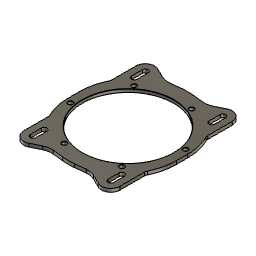
Motor_Base_Plate_Top v5 (Autodesk Fusion 360 archive; units mm, degrees)
design "Motor_Base_Plate_Top v5" references "Forged Hexagon Socket Head Cap Screw ANSI B18.3.1M - M4x0.7 x 6 Steel Grade 2 Plain"
Autodesk Fusion 360 part; units mm, degrees
sketch "Sketch1" plane through (0, 0, 0) normal (0, 0, 1) x (1, 0, 0)
  line L0 (0, 0) -> (42.0984, 0) construction
  line L1 (0, 2.5) -> (0, 20)
  line L2 (20, 0) -> (2.5, 0)
  line L3 (43.5453, 45.7571) -> (43.5453, 28.6506)
  arc A0 (32.6927, 46.2539) -> (32.6429, 45.7571) centre (35.1429, 45.7571) ccw
  line L4 (-32.6429, 45.7571) -> (-32.6429, 40.7571)
  arc A1 (-32.6429, 45.7571) -> (-32.7077, 46.3226) centre (-35.1429, 45.7571) ccw
  line L5 (-43.5453, 45.7571) -> (-43.5453, 28.6506)
  line L6 (16.6515, 53.2283) -> (16.6515, 59.0493) construction
  line L7 (-15.557, 53.706) -> (-15.557, 59.527) construction
  line L8 (0, 0) -> (45, 0) construction
  arc A2 (-41.8537, 25.4807) -> (-42.1265, 25.0272) centre (0, 0) ccw
  arc A3 (4.0267, 61.4469) -> (-4.7848, 61.3754) centre (-0.036, 19.1415) ccw
  arc A4 (43.4103, 49.257) -> (33.6006, 59.0168) centre (35.1429, 50.7571) ccw
  line L9 (16.6515, 58.2283) -> (16.6515, 64.0493) construction
  arc A5 (28.1023, 59.5419) -> (33.6006, 59.0168) centre (31.7651, 68.8469) ccw
  arc A6 (14.9315, 52.7652) -> (22.9245, 54.1858) centre (16.401, 67.693) ccw
  line L10 (-22.9245, 54.1858) -> (-31.3596, 58.2597)
  arc A7 (49, 5) -> (41.8537, 30.4807) centre (0, 5) ccw
  line L11 (43.5453, 50.7571) -> (43.5453, 28.6506)
  line L12 (14.9315, 52.7652) -> (5.4274, 53.7007)
  line L13 (-41.2861, 38.5638) -> (-43.4103, 49.257)
  arc A8 (-9.7818, 62.096) -> (-4.7848, 61.3754) centre (-5.9022, 71.3127) ccw
  line L14 (-14.9315, 52.7652) -> (-5.4274, 53.7007)
  arc A9 (-37.6429, 40.7571) -> (-32.6429, 40.7571) centre (-35.1429, 40.7571) ccw
  circle A10 centre (-15.557, 58.706) radius 1.5
  line L15 (-43.5453, 50.7571) -> (-43.5453, 28.6506)
  arc A11 (-44.0504, 26.4608) -> (-43.5453, 28.6506) centre (-48.5453, 28.6506) ccw
  arc A12 (-32.6429, 50.7571) -> (-37.6429, 50.7571) centre (-35.1429, 50.7571) ccw
  line L16 (-19.3563, 63.0202) -> (-28.095, 59.5544)
  arc A13 (-33.6082, 59.0182) -> (-28.095, 59.5544) centre (-31.7817, 68.85) ccw
  line L17 (-7.2407, 61.0264) -> (-0.4717, 58.2301) construction
  arc A14 (-11.79, 62.9413) -> (-19.3563, 63.0202) centre (-15.6696, 53.7246) ccw
  arc A15 (43.5453, 28.6506) -> (44.0504, 26.4608) centre (48.5453, 28.6506) ccw
  line L18 (-11.79, 62.9413) -> (-9.7818, 62.096)
  line L19 (41.2861, 38.5638) -> (43.4103, 49.257)
  arc A16 (-7.2407, 61.0264) -> (6.4194, 61.1484) centre (-0.036, 19.1415) ccw construction
  line L20 (-32.6429, 50.7571) -> (-32.6429, 45.7571)
  arc A17 (-22.9245, 54.1858) -> (-14.9315, 52.7652) centre (-16.401, 67.693) ccw
  arc A18 (41.2861, 38.5638) -> (41.8537, 30.4807) centre (56.0268, 35.5374) ccw
  line L21 (-15.557, 58.706) -> (-15.557, 64.527) construction
  line L22 (11.1293, 63.1457) -> (8.8867, 62.1947)
  arc A19 (4.0267, 61.4469) -> (8.8867, 62.1947) centre (4.9826, 71.4011) ccw
  line L23 (6.4194, 61.1484) -> (-0.4717, 58.2301) construction
  arc A20 (43.4103, 49.257) -> (31.3596, 58.2597) centre (35.1429, 50.7571) ccw
  line L24 (-37.6429, 50.7571) -> (-37.6429, 40.7571)
  arc A21 (-33.6006, 59.0168) -> (-43.4103, 49.257) centre (-35.1429, 50.7571) ccw
  arc A22 (-41.8537, 30.4807) -> (-41.2861, 38.5638) centre (-56.0268, 35.5374) ccw
  arc A23 (-31.3596, 58.2597) -> (-43.4103, 49.257) centre (-35.1429, 50.7571) ccw
  arc A24 (18.6963, 63.2444) -> (11.1293, 63.1457) centre (15.0335, 53.9393) ccw
  arc A25 (5.4274, 53.7007) -> (-5.4274, 53.7007) centre (0, 5) ccw
  circle A26 centre (16.6515, 58.2283) radius 1.5
  arc A27 (-41.8537, 30.4807) -> (-49, 5) centre (0, 5) ccw
  line L25 (18.6963, 63.2444) -> (28.1023, 59.5419)
  line L26 (22.9245, 54.1858) -> (31.3596, 58.2597)
  arc A28 (-33.6006, 54.0168) -> (-33.6082, 54.0182) centre (-35.1429, 45.7571) ccw
  line L27 (32.6429, 45.7571) -> (32.6429, 40.7571)
  line L28 (32.6429, 50.7571) -> (32.6429, 45.7571)
  line L29 (37.6429, 50.7571) -> (37.6429, 40.7571)
  arc A29 (37.6429, 50.7571) -> (32.6429, 50.7571) centre (35.1429, 50.7571) ccw
  arc A30 (32.6429, 40.7571) -> (37.6429, 40.7571) centre (35.1429, 40.7571) ccw
  arc A31 (-5.4274, -53.7007) -> (5.4274, -53.7007) centre (0, -5) ccw
  arc A32 (22.9245, -54.1858) -> (14.9315, -52.7652) centre (16.401, -67.693) ccw
  arc A33 (32.6429, -45.7571) -> (32.6927, -46.2539) centre (35.1429, -45.7571) ccw
  line L30 (-15.557, -53.706) -> (-15.557, -59.527) construction
  arc A34 (31.3596, -58.2597) -> (43.4103, -49.257) centre (35.1429, -50.7571) ccw
  line L31 (6.4194, -61.1484) -> (-0.4717, -58.2301) construction
  circle A35 centre (16.6515, -58.2283) radius 1.5
  arc A36 (-49, -5) -> (-41.8537, -30.4807) centre (0, -5) ccw
  arc A37 (32.6429, -50.7571) -> (37.6429, -50.7571) centre (35.1429, -50.7571) ccw
  arc A38 (-42.1265, -25.0272) -> (-41.8537, -25.4807) centre (0, 0) ccw
  line L32 (-11.79, -62.9413) -> (-9.7818, -62.096)
  arc A39 (8.8867, -62.1947) -> (4.0267, -61.4469) centre (4.9826, -71.4011) ccw
  arc A40 (-41.2861, -38.5638) -> (-41.8537, -30.4807) centre (-56.0268, -35.5374) ccw
  line L33 (11.1293, -63.1457) -> (8.8867, -62.1947)
  arc A41 (-43.5453, -28.6506) -> (-44.0504, -26.4608) centre (-48.5453, -28.6506) ccw
  line L34 (-22.9245, -54.1858) -> (-31.3596, -58.2597)
  arc A42 (-19.3563, -63.0202) -> (-11.79, -62.9413) centre (-15.6696, -53.7246) ccw
  arc A43 (-33.6082, -54.0182) -> (-33.6006, -54.0168) centre (-35.1429, -45.7571) ccw
  arc A44 (-37.6429, -50.7571) -> (-32.6429, -50.7571) centre (-35.1429, -50.7571) ccw
  arc A45 (-4.7848, -61.3754) -> (4.0267, -61.4469) centre (-0.036, -19.1415) ccw
  arc A46 (-32.7077, -46.3226) -> (-32.6429, -45.7571) centre (-35.1429, -45.7571) ccw
  line L35 (-32.6429, -45.7571) -> (-32.6429, -40.7571)
  line L36 (22.9245, -54.1858) -> (31.3596, -58.2597)
  line L37 (-15.557, -58.706) -> (-15.557, -64.527) construction
  line L38 (32.6429, -45.7571) -> (32.6429, -40.7571)
  line L39 (32.6429, -50.7571) -> (32.6429, -45.7571)
  line L40 (-43.5453, -45.7571) -> (-43.5453, -28.6506)
  line L41 (37.6429, -50.7571) -> (37.6429, -40.7571)
  line L42 (14.9315, -52.7652) -> (5.4274, -53.7007)
  arc A47 (-14.9315, -52.7652) -> (-22.9245, -54.1858) centre (-16.401, -67.693) ccw
  line L43 (43.5453, -45.7571) -> (43.5453, -28.6506)
  line L44 (-43.5453, -50.7571) -> (-43.5453, -28.6506)
  arc A48 (-43.5453, -23.6506) -> (-44.0504, -21.4608) centre (-48.5453, -23.6506) ccw
  line L45 (41.2861, -38.5638) -> (43.4103, -49.257)
  arc A49 (-28.095, -59.5544) -> (-33.6082, -59.0182) centre (-31.7817, -68.85) ccw
  arc A50 (-4.7848, -61.3754) -> (-9.7818, -62.096) centre (-5.9022, -71.3127) ccw
  line L46 (20, 0) -> (2.5, 0)
  line L47 (16.6515, -53.2283) -> (16.6515, -59.0493) construction
  line L48 (18.6963, -63.2444) -> (28.1023, -59.5419)
  arc A51 (33.6006, -59.0168) -> (43.4103, -49.257) centre (35.1429, -50.7571) ccw
  line L49 (-7.2407, -61.0264) -> (-0.4717, -58.2301) construction
  arc A52 (41.8537, -30.4807) -> (49, -5) centre (0, -5) ccw
  arc A53 (-43.4103, -49.257) -> (-33.6006, -59.0168) centre (-35.1429, -50.7571) ccw
  line L50 (16.6515, -58.2283) -> (16.6515, -64.0493) construction
  arc A54 (44.0504, -26.4608) -> (43.5453, -28.6506) centre (48.5453, -28.6506) ccw
  circle A55 centre (-15.557, -58.706) radius 1.5
  line L51 (-41.2861, -38.5638) -> (-43.4103, -49.257)
  arc A56 (41.8537, -30.4807) -> (41.2861, -38.5638) centre (56.0268, -35.5374) ccw
  arc A57 (33.6006, -59.0168) -> (28.1023, -59.5419) centre (31.7651, -68.8469) ccw
  line L52 (-19.3563, -63.0202) -> (-28.095, -59.5544)
  line L53 (-37.6429, -50.7571) -> (-37.6429, -40.7571)
  arc A58 (6.4194, -61.1484) -> (-7.2407, -61.0264) centre (-0.036, -19.1415) ccw construction
  line L54 (-14.9315, -52.7652) -> (-5.4274, -53.7007)
  line L55 (-32.6429, -50.7571) -> (-32.6429, -45.7571)
  arc A59 (37.6429, -40.7571) -> (32.6429, -40.7571) centre (35.1429, -40.7571) ccw
  arc A60 (-43.4103, -49.257) -> (-31.3596, -58.2597) centre (-35.1429, -50.7571) ccw
  arc A61 (-32.6429, -40.7571) -> (-37.6429, -40.7571) centre (-35.1429, -40.7571) ccw
  line L56 (43.5453, -50.7571) -> (43.5453, -28.6506)
  arc A62 (11.1293, -63.1457) -> (18.6963, -63.2444) centre (15.0335, -53.9393) ccw
  line L57 (49, 5) -> (49, -5)
  line L58 (-49, -5) -> (-49, 5)
  circle A63 centre (0, 0) radius 45 construction
  line L59 (0, 0) -> (45, 0) construction
  circle A64 centre (0, 0) radius 41.25
  line L60 (0, 0) -> (45, 0) construction
  line L61 (0, 0) -> (45, 0) construction
  line L62 (0, 0) -> (45, 0) construction
  line L63 (0, 0) -> (-15.3909, -42.2862) construction
  line L64 (0, 0) -> (45, 0) construction
  circle A65 centre (-15.3909, -42.2862) radius 2
  circle A66 centre (28.9254, -34.472) radius 2
  circle A67 centre (44.3163, 7.8142) radius 2
  circle A68 centre (15.3909, 42.2862) radius 2
  circle A69 centre (-28.9254, 34.472) radius 2
  circle A70 centre (-44.3163, -7.8142) radius 2
  point P0 (0, 5)
  point P1 (0, 5)
  point P2 (0, -5)
  point P3 (0, -2.5)
  point P4 (0, -5)
  point P5 (42.0984, 0)
  point P6 (0, -20)
  point P7 (45, 0)
  dimension "d52" = 5.821
  dimension "d53" = 5.821
  dimension "d60" = 85
  dimension "d61" = 3
  dimension "d62" = 5.821
  dimension "d63" = 5.821
  dimension "d64" = 10
  dimension "d66" = 90
  dimension "d71" = 82.5
  dimension "d121" = 110
  dimension "d122" = 4
  dimension "d124" = 360
  constraint coincident L0.start L8.start
  constraint horizontal L0
  constraint symmetric L1 L3.start L5.start
  constraint vertical L6
  constraint vertical L7
  constraint horizontal L8
  constraint tangent L14 A17
  constraint concentric A25 A27
  constraint coincident L9.start A16
  constraint coincident A10.centre A16
  constraint coincident L9.start A26.centre
  constraint vertical L9
  constraint coincident A10.centre L21.start
  constraint vertical L21
  constraint concentric A3 A16
  constraint coincident A20.end L25
  constraint coincident A20.end A4
  constraint tangent A4 A5
  constraint tangent A5 L25
  constraint coincident L9.end L25
  constraint tangent A24 L25
  constraint tangent L22 A24
  constraint equal A5 A24
  constraint coincident A16.end L22
  constraint tangent L22 A19
  constraint tangent A3 A19
  constraint equal A5 A19
  constraint coincident L17.start L18
  constraint coincident L17.start A3
  constraint tangent A3 A8
  constraint tangent A8 L18
  constraint equal A5 A8
  constraint coincident L21.end L16
  constraint coincident L21.end L18
  constraint tangent L16 A14
  constraint tangent A14 L18
  constraint equal A5 A14
  constraint tangent L16 A13
  constraint equal A5 A13
  constraint coincident A16 A2.end
  constraint coincident A16 A1.end
  constraint coincident A16 A0.start
  constraint symmetric L1 L4.start A0.end
  constraint symmetric L1 A12.start L28.start
  constraint symmetric L1 A12.end L29.start
  constraint symmetric L1 L4.end L27.end
  constraint symmetric L1 A9.start L29.end
  constraint symmetric L1 A9 A30
  constraint symmetric L1 A12 A29
  constraint symmetric L8.start L0 A2.centre
  constraint symmetric P5 L0 L0.end
  constraint symmetric L0 L8.start A2.centre
  constraint symmetric L0 A2.start A38.end
  constraint symmetric L0 L1.start P3
  constraint symmetric L0 L1.end P6
  constraint symmetric L0 L2.start L46.start
  constraint symmetric L0 L2.end L46.end
  constraint symmetric L0 L3.start L43.start
  constraint symmetric L0 A0.end A33.start
  constraint symmetric L0 A0 A33
  constraint symmetric L0 L4.start A46.end
  constraint symmetric L0 A1 A46
  constraint symmetric L0 L5.start L40.start
  constraint symmetric L0 L6.start L47.start
  constraint symmetric L0 L6.end L47.end
  constraint symmetric L0 L7.start L30.start
  constraint symmetric L0 L7.end L30.end
  constraint symmetric L0 A28.end A43.start
  constraint symmetric L0 A28.start A43.end
  constraint symmetric L0 P7 L8.end
  constraint symmetric L0 A2 A38
  constraint symmetric L0 L9.end L50.end
  constraint symmetric L0 P1 P4
  constraint symmetric L0 L12.end A31.end
  constraint symmetric L0 L13.start A40.start
  constraint symmetric L0 A15.end A54.start
  constraint symmetric L0 A4.end A51.start
  constraint symmetric L0 A4.start A34.end
  constraint symmetric L0 A12.start A44.end
  constraint symmetric L0 A12.end A44.start
  constraint symmetric L0 L9.start A35.centre
  constraint symmetric L0 L4.end L35.end
  constraint symmetric L0 L22.start L33.start
  constraint symmetric L0 A16.end L31.start
  constraint symmetric L0 L19.start L45.start
  constraint symmetric L0 A20.end A34.start
  constraint symmetric L0 A7.end A52.start
  constraint symmetric L0 A3.start A39.end
  constraint symmetric L0 L22.end A39.start
  constraint symmetric L0 A6.end A32.start
  constraint symmetric L0 L10.start L34.start
  constraint symmetric L0 A24.start L48.start
  constraint symmetric L0 L15.start L44.start
  constraint symmetric L0 A3.end A45.start
  constraint symmetric L0 L10.end L34.end
  constraint symmetric L0 L5.end A41.start
  constraint symmetric L0 L13.end A53.start
  constraint symmetric L0 A7.start A52.end
  constraint symmetric L0 A5.start L48.end
  constraint symmetric L0 A11.start A41.end
  constraint symmetric L0 L14.end A31.start
  constraint symmetric L0 L17.start L49.start
  constraint symmetric L0 A21.start A53.end
  constraint symmetric L0 L21.end L37.end
  constraint symmetric L0 A10.centre L37.start
  constraint symmetric L0 L3.end L43.end
  constraint symmetric L0 L16.start A42.start
  constraint symmetric L0 A8.start L32.end
  constraint symmetric L0 A14.start L32.start
  constraint symmetric L0 A9.start L53.end
  constraint symmetric L0 A22.start A36.end
  constraint symmetric L0 A6.start A32.end
  constraint symmetric L0 L16.end A49.start
  constraint symmetric L0 L11.start L56.start
  constraint symmetric L0 A27.end A36.start
  constraint symmetric L0 L14.start A47.start
  constraint symmetric L0 L17.end L31.end
  constraint symmetric L0 A13.start A49.end
  constraint symmetric L0 A3 A45
  constraint symmetric L0 A4 A51
  constraint symmetric L0 A5 A57
  constraint symmetric L0 A6 A32
  constraint symmetric L0 A7 A52
  constraint symmetric L0 A8 A50
  constraint symmetric L0 A9 A61
  constraint symmetric L0 A10 A55
  constraint symmetric L0 A11 A41
  constraint symmetric L0 A12 A44
  constraint symmetric L0 A13 A49
  constraint symmetric L0 A14 A42
  constraint symmetric L0 A15 A54
  constraint symmetric L0 A16 A58
  constraint symmetric L0 A17 A47
  constraint symmetric L0 A18 A56
  constraint symmetric L0 A19 A39
  constraint symmetric L0 A20 A34
  constraint symmetric L0 A21 A53
  constraint symmetric L0 A22 A40
  constraint symmetric L0 A23 A60
  constraint symmetric L0 A24 A62
  constraint symmetric L0 A25 A31
  constraint symmetric L0 A26 A35
  constraint symmetric L0 A27 A36
  constraint symmetric L0 A2.end A38.start
  constraint symmetric L0 A28 A43
  constraint symmetric L0 A1.end A46.start
  constraint symmetric L0 A0.start A33.end
  constraint symmetric L0 L27.end L38.end
  constraint symmetric L0 L28.start A37.start
  constraint symmetric L0 L29.start A37.end
  constraint symmetric L0 L29.end L41.end
  constraint symmetric L0 A29 A37
  constraint symmetric L0 A30 A59
  constraint tangent A52 L57
  constraint tangent A27 L58
  constraint horizontal L59
  constraint concentric A2 A64
  constraint horizontal L60
  constraint horizontal L61
  constraint horizontal L62
  constraint horizontal L64
  constraint coincident L63.end A65.centre
  measures "d52" distance of L6.start L6.end
  measures "d53" distance of L7.start L7.end
  measures "d60" diameter of A16
  measures "d61" diameter of A26
  measures "d62" distance of L9.end L9.start
  measures "d63" distance of L21.end A10.centre
  measures "d64" radius of A5
  measures "d66" diameter of A63
  measures "d71" diameter of A64
  measures "d121" angle of L63 L64
  measures "d122" diameter of A65
extrude "Extrude1" add sketch "Sketch1" along normal blind 3 contours L3 A4 A7 L11 A15 L19 A18 A20 | A4 A6 L10 A7 L12 L13 L14 A13 L19 A17 A18 A20 A21 A22 A23 A25 A27 L26 A31 A32 A34 A36 A40 L34 L36 L42 A47 L45 A49 A51 A52 A53 L51 A56 L54 A60 L57 L58 | A34 L43 L45 A51 A52 A54 A56 L56 | L5 L13 L15 A11 A21 A22 A23 A27 | A36 A40 A41 L40 L44 A53 L51 A60
chamfer "Chamfer1" distance 0.25 angle 45 1 faces at (-41.045, -4.1072, 1)
chamfer "Chamfer1" distance 0.25 angle 45 6 faces at (30.923, -34.5717, 2) (-13.3934, -42.3859, 2) (-42.3188, -7.9139, 2) (46.3139, 7.7145, 2) (-26.9279, 34.3723, 2) (17.3884, 42.1865, 2)
thread "Thread7" [rolled back] thread offset 0 thread length 10
other "Screw1"
other "Screw2"
other "Screw3"
other "Screw4"
other "Screw5"
other "Screw6"
equation "d121 = 90 deg + 20 deg"

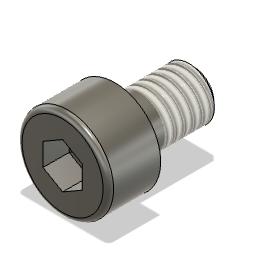
design "Forged Hexagon Socket Head Cap Screw ANSI B18.3.1M - M4x0.7 x 6 Steel Grade 2 Plain"
description: Forged Hexagon Socket Head Cap Screw ANSI B18.3.1M - M4x0.7 x 6
Autodesk Fusion 360 part; units mm, degrees
sketch "Sketch1" plane through (0, 0, 0) normal (0, 1, 0) x (1, 0, 0)
  line L0 (-2, 0) -> (-2, 6)
  line L1 (-2, 6) -> (0, 6)
  line L2 (0, 6) -> (0, -4)
  line L3 (-2, 0) -> (-3.5, 0)
  line L4 (-3.5, 0) -> (-3.5, -4)
  line L5 (-3.5, -4) -> (0, -4)
  dimension "d9" = 4
  dimension "d66" = 7
  dimension "d68" = 6
  dimension "d79" = 4
  constraint perpendicular L0 L1
  constraint collinear origin L1.end L2.end
  constraint perpendicular L0 L3
  constraint coincident origin L3
  constraint vertical L0
  constraint vertical L2
  constraint parallel L2 L4
  constraint coincident L2 L5.end
  constraint perpendicular L2 L5
  measures "d68" distance of origin L1.end
  measures "d79" distance of L3.end L4.end
revolve "Revolve1" add sketch "Sketch1" angle 360 about axis through (0, 0, -6) along (0, 0, 1)
ref_plane "WorkPlane1" through (0, 0, 4) normal (0, 0, 1) x (1, 0, 0)
sketch "Sketch6" plane through (0, 0, 4) normal (0, 0, 1) x (1, 0, 0)
  line L0 (-1.5, 0) -> (1.5, 0) construction
  line L1 (0, 0) -> (-1.5, 0.866)
  line L2 (-1.5, -0.866) -> (-1.5, 0.866)
  line L3 (-1.5, -0.866) -> (0, 0)
  dimension "d72" = 3
  dimension "d100" = 150
  constraint horizontal L0
  constraint midpoint L1.start L0
  constraint coincident L1.start L3.end
  constraint perpendicular L0 L2
  constraint midpoint L0.start L2
  constraint coincident L1.end L2.end
  measures "d72" distance of L0.start L0.end
  measures "d100" angle of L0 L1
extrude "Extrude1" cut sketch "Sketch6" against normal blind 2
pattern_circular "C-Pattern1" count 6 over 360 about axis through (0, 0, 1.75) along (0, 0, 1) of "Extrude1"
extrude "Extrude2" cut 1 faces at (0, -0.5774, 2) along direction (0, 0, -1) blind 2 draft -85
thread "Thread2" "ANSI Metric M Profile 4.0 M4x0.7 4g6g" major diameter 3.908 minor diameter 3.128 pitch 0.7 angle 60 resizes the face on face at (-1.9975, 0.0997, -2) from (0, 0, -1.8294) to (0, 0, -6)
fillet "Fillet4" radius 0.4 1 edges at (-3.2631, 1.2657, 4)
sketch "Sketch7" plane through (0, 0, 0) normal (0, 1, 0) x (1, 0, 0)
  line L0 (-2.04, 6) -> (-2.04, 5.5706)
  line L1 (-2.04, 5.5706) -> (-1.5706, 6)
  line L2 (0, 6) -> (0, -4)
  line L3 (-2.04, 6) -> (0, 6)
  dimension "d92" = 0.4294
  dimension "d98" = 1.5706
  dimension "d99" = 2.04
  constraint coincident L2.start L3.end
  constraint perpendicular L2 L3
  constraint coincident L1.end L3
  constraint perpendicular L0 L3
  measures "d92" vertical distance of L0.end L1.end
  measures "d98" horizontal distance of origin L1.end
  measures "d99" distance of origin L0
revolve "Revolve3" cut sketch "Sketch7" angle 360 about axis through (0, 0, 1.75) along (0, 0, 1)
equation "d9 = adsk_nomdia"
equation "adsk_nomlen = 6.00 mm"
equation "adsk_headh = 4.00 mm"
equation "adsk_headdia = 7.00 mm"
equation "adsk_nomdia = 4.00 mm"
equation "adsk_philwidth = 3.00 mm"
equation "d31 = -adsk_phildepth"
equation "adsk_phildepth = 2.00 mm"
equation "d66 = adsk_headdia"
equation "d68 = adsk_nomlen"
equation "d71 = adsk_headh"
equation "d72 = adsk_philwidth"
equation "d76 = -adsk_phildepth"
equation "d79 = adsk_headh"
equation "adsk_thrlen = 4.170585 mm"
equation "d84 = adsk_thrlen"
equation "d86 = adsk_nomdia * 0.1"
equation "d92 = adsk_startlen"
equation "adsk_startlen = 0.429415 mm"
equation "adsk_endpointdia = 3.14117 mm"
equation "d98 = adsk_endpointdia / 2"
equation "d99 = adsk_nomdia * 0.51"
